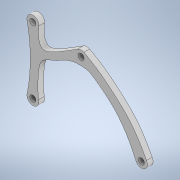
# Autodesk Inventor part: Bracket Concept MK3
Saved by Autodesk Inventor 2021 (Build 250183000, 183)
## iProperties
Created: 2021-05-11
Part Number: Bracket Concept MK3
Material: Generic
Document SubType Name: Modeling
Designer: Jawal
Density: 1 g/cm^3
Appearance: Default
Author: Jawal
Autodesk Inventor part; units mm, degrees
ref_plane "YZ Plane" through (0, 0, 0) normal (1, 0, 0) x (0, 1, 0)
ref_plane "XZ Plane" through (0, 0, 0) normal (0, 1, 0) x (-1, 0, 0)
ref_plane "XY Plane" through (0, 0, 0) normal (0, 0, 1) x (1, 0, 0)
sketch "Sketch1" plane through (0, 0, 0) normal (0, 0, 1) x (1, 0, 0)
  line L0 (-110, 70) -> (110, 70) construction
  line L1 (110, 70) -> (110, -70) construction
  line L2 (110, -70) -> (-110, -70) construction
  line L3 (-110, -70) -> (-110, 70) construction
  circle A0 centre (-90, 55) radius 5
  circle A1 centre (-90, -55) radius 5
  circle A2 centre (90, -55) radius 5
  circle A3 centre (-10, 45) radius 5
  line L4 (-67, 0) -> (-42, 0) construction
  line L5 (-42, 0) -> (-42, -30) construction
  line L6 (-42, -30) -> (-67, -30) construction
  line L7 (-67, -30) -> (-67, 0) construction
  circle A4 centre (-54.5, -11) radius 10 construction
  circle A5 centre (-63.5044, -24.4163) radius 3 construction
  circle A6 centre (-57.3559, -26.4695) radius 3 construction
  circle A7 centre (-51.263, -24.6531) radius 3 construction
  circle A8 centre (-45.3418, -26.5938) radius 3 construction
  arc A9 (-80.0339, 54.177) -> (-99.4444, 51.7131) centre (-90, 55) ccw
  arc A10 (80.256, -57.2483) -> (98.4155, -49.5982) centre (90, -55) ccw
  arc A11 (-99.4444, -51.7131) -> (-80.5128, -51.8388) centre (-90, -55) ccw
  arc A12 (-5.3594, 53.858) -> (-16.2673, 52.7923) centre (-10, 45) ccw
  line L8 (-99.4444, 51.7131) -> (-95, 27.4878) construction
  line L9 (-95, 27.4878) -> (-93.8149, 3.2662) construction
  line L10 (-93.8149, 3.2662) -> (-93.8149, -21) construction
  line L11 (-93.8149, -21) -> (-97.9589, -43.6087) construction
  line L12 (-97.9589, -43.6087) -> (-99.4444, -51.7131) construction
  spline S0 degree 4 poles (-99.4444, 51.7131) (-95, 27.4878) (-93.8149, 3.2662) (-93.8149, -21) (-97.9589, -43.6087) (-99.4444, -51.7131) knots 1 1 1 1 1 2 3 3 3 3 3
  line L13 (-80.0339, 54.177) -> (-80.9917, 42.5781) construction
  line L14 (-80.9917, 42.5781) -> (-80.9917, 31.0335) construction
  line L15 (-80.9917, 31.0335) -> (-74.3239, 18.9012) construction
  line L16 (-74.3239, 18.9012) -> (-58.5299, 25.7807) construction
  line L17 (-58.5299, 25.7807) -> (-18.4474, 51.5962) construction
  line L18 (-18.4474, 51.5962) -> (-16.2673, 52.7923) construction
  spline S1 degree 4 poles (-80.0339, 54.177) (-80.9917, 42.5781) (-80.9917, 31.0335) (-74.3239, 18.9012) (-58.5299, 25.7807) (-18.4474, 51.5962) (-16.2673, 52.7923) knots 1 1 1 1 1 2 3 4 4 4 4 4
  line L19 (-80.5128, -51.8388) -> (-81.9566, -43.6087) construction
  line L20 (-81.9566, -43.6087) -> (-81.9566, -21) construction
  line L21 (-81.9566, -21) -> (-80.5128, 3.2662) construction
  line L22 (-80.5128, 3.2662) -> (-70.6976, 12.3031) construction
  line L23 (-70.6976, 12.3031) -> (-51.263, 17.488) construction
  line L24 (-51.263, 17.488) -> (-30.2965, 32.65) construction
  line L25 (-30.2965, 32.65) -> (-8.3751, 32.65) construction
  line L26 (-8.3751, 32.65) -> (5.2827, 31.0335) construction
  line L27 (5.2827, 31.0335) -> (14.5834, 22.3409) construction
  line L28 (14.5834, 22.3409) -> (59.8169, -8.8669) construction
  line L29 (59.8169, -8.8669) -> (77.6071, -52.4205) construction
  line L30 (77.6071, -52.4205) -> (80.256, -57.2483) construction
  spline S2 degree 4 poles (-80.5128, -51.8388) (-81.9566, -43.6087) (-81.9566, -21) (-80.5128, 3.2662) (-70.6976, 12.3031) (-51.263, 17.488) (-30.2965, 32.65) (-8.3751, 32.65) (5.2827, 31.0335) (14.5834, 22.3409) (59.8169, -8.8669) (77.6071, -52.4205) (80.256, -57.2483) knots 1 1 1 1 1 2 3 4 5 6 7 8 9 10 10 10 10 10
  line L31 (-5.3594, 53.858) -> (9.6288, 46.0058) construction
  line L32 (9.6288, 46.0058) -> (31.8174, 31.0335) construction
  line L33 (31.8174, 31.0335) -> (59.8169, 6.737) construction
  line L34 (59.8169, 6.737) -> (80, -15) construction
  line L35 (80, -15) -> (98.4155, -49.5982) construction
  spline S3 degree 4 poles (-5.3594, 53.858) (9.6288, 46.0058) (31.8174, 31.0335) (59.8169, 6.737) (80, -15) (98.4155, -49.5982) knots 1 1 1 1 1 2 3 3 3 3 3
  point P0 (0, 0)
  dimension "d1" = 70
  dimension "d2" = 70
  dimension "d3" = 110
  dimension "d4" = 110
  dimension "d5" = 10
  dimension "d6" = 10
  dimension "d7" = 10
  dimension "d8" = 10
  dimension "d9" = 55
  dimension "d10" = 55
  dimension "d11" = 55
  dimension "d12" = 180
  dimension "d13" = 90
  dimension "d14" = 90
  dimension "d16" = 45
  dimension "d17" = 42
  dimension "d18" = 30
  dimension "d19" = 0
  dimension "d20" = 25
  dimension "d21" = 20
  dimension "d22" = 6
  dimension "d23" = 6
  dimension "d24" = 6
  dimension "d25" = 11
  dimension "d26" = 12.5
  dimension "d27" = 6
  dimension "d41" = 20
  dimension "d43" = 20
  dimension "d44" = 20
  dimension "d45" = 20
  dimension "d46" = 10
  constraints: 16 end point, 13 centre point, 8 point on circle, 4 coincident, 4 parallel, 3 horizontal, 3 perpendicular, 2 tangent, 2 vertical, 12 other
  measures "d1" distance from line of point (0, 0) L2
  measures "d2" distance from line of point (0, 0) L0
  measures "d3" distance from line of L1 point (0, 0)
  measures "d4" distance from line of point (0, 0) L3
  measures "d5" diameter of A0
  measures "d6" diameter of A1
  measures "d7" diameter of A2
  measures "d8" diameter of A3
  measures "d9" vertical distance of point (0, 0) A0.centre
  measures "d10" vertical distance of point (0, 0) A1.centre
  measures "d11" vertical distance of A2.centre point (0, 0)
  measures "d12" distance of A2.centre A1.centre
  measures "d13" horizontal distance of point (0, 0) A0.centre
  measures "d14" horizontal distance of point (0, 0) A1.centre
  measures "d16" vertical distance of point (0, 0) A3.centre
  measures "d17" distance from line of point (0, 0) L5
  measures "d18" distance of L4.end L5.end
  measures "d19" distance from line of L4 point (0, 0)
  measures "d20" distance of L5.end L6.end
  measures "d21" diameter of A4
  measures "d22" diameter of A5
  measures "d23" diameter of A6
  measures "d24" diameter of A7
  measures "d25" distance from line of L4 A4.centre
  measures "d26" distance from line of L7 A4.centre
  measures "d27" diameter of A8
  measures "d41" diameter of A9
  measures "d43" diameter of A10
  measures "d44" diameter of A11
  measures "d45" diameter of A12
  measures "d46" horizontal distance of point (0, 0) A3.centre
extrude "Extrusion3" add sketch "Sketch1" along normal blind 9.4
equation "\"d1\" = d2"
equation "\"d4\" = d3"
equation "\"d10\" = d9"
equation "\"d11\" = d9"
equation "\"d14\" = d13"
equation "\"d26\" = 0.5 * d20"
body "Solid3"
